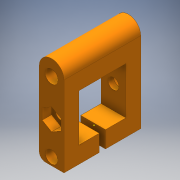
# Autodesk Inventor part: arm_grip
Saved by Autodesk Inventor 2016 (Build 200138000, 138)
## iProperties
Created: 2016-09-22
Part Number: arm_grip
Material: Nylon 6/6
Document SubType Name: Modeling
Designer: Jakub
Density: 1.13 g/cm^3
Appearance: Nylon 6
Mass: 4.12731 g
Surface Area: 27.5529 cm^2
Volume: 3.65248 cm^3
Author: Jakub
Autodesk Inventor part; units mm, degrees
ref_plane "YZ Plane" through (0, 0, 0) normal (1, 0, 0) x (0, 1, 0)
ref_plane "XZ Plane" through (0, 0, 0) normal (0, 1, 0) x (-1, 0, 0)
ref_plane "XY Plane" through (0, 0, 0) normal (0, 0, 1) x (1, 0, 0)
sketch "Sketch1" plane through (0, 0, 0) normal (1, 0, 0) x (0, 1, 0)
  line L0 (-12.4, 15) -> (12.4, 15)
  line L1 (12.4, 15) -> (12.4, -15)
  line L2 (12.4, -15) -> (-12.4, -15)
  line L3 (-12.4, -15) -> (-12.4, 15)
  line L4 (-12.4, 15) -> (12.4, -15) construction
  line L5 (12.4, 15) -> (-12.4, -15) construction
  line L6 (0, -15) -> (0, -1.5)
  circle A0 centre (0, -1.5) radius 8
  point P0 (0, 0)
  dimension "d0" = 24.8
  dimension "d1" = 30
  dimension "d2" = 13.5
  dimension "d3" = 16
  constraints: 14 end point, 3 midpoint, 2 parallel, 1 centre point, 1 coincident, 1 horizontal, 1 perpendicular, 1 vertical
  measures "d0" distance of L1.end L2.end
  measures "d1" distance of L0.end L1.end
  measures "d2" distance of L6.start L6.end
  measures "d3" diameter of A0
extrude "Extrusion1" add sketch "Sketch1" along normal blind 8
sketch "Sketch3" plane through (0, 12.4, 15) normal (0, 1, 0) x (1, 0, 0)
  line L0 (0, 0) -> (8, 0) projected
  line L1 (4, 0) -> (4, 5)
  circle A0 centre (4, 5) radius 2.1
  point P0 (0, 15)
  dimension "d9" = 5
  dimension "d10" = 4.2
  constraints: 2 end point, 1 centre point, 1 coincident, 1 midpoint, 1 vertical
  measures "d9" distance of L1.start L1.end
  measures "d10" diameter of A0
extrude "Extrusion3" cut sketch "Sketch3" against normal up to next
sketch "Sketch4" plane through (0, 12.4, 15) normal (0, 1, 0) x (1, 0, 0)
  line L0 (0, 30) -> (8, 30) projected
  line L1 (4, 30) -> (4, 27.5)
  circle A0 centre (4, 27.5) radius 1.25
  point P0 (0, 15)
  dimension "d13" = 2.5
  dimension "d14" = 2.5
  constraints: 2 end point, 1 centre point, 1 coincident, 1 midpoint, 1 vertical
  measures "d13" distance of L1.start L1.end
  measures "d14" diameter of A0
extrude "Extrusion4" cut sketch "Sketch4" against normal through all
fillet "Fillet1" radius 4 2 edges at (0, 0, 15) (8, 0, 15)
fillet "Fillet2" radius 2 1 edges at (0, 0, -15)
sketch "Sketch5" plane through (8, 0, 0) normal (1, 0, 0) x (0, 0, -1)
  arc A0 (1.5, 8) -> (1.5, 8) centre (1.5, 0) ccw projected
  circle A1 centre (1.5, 0) radius 8
  point P0 (0, 0)
  constraints: 1 centre point, 1 coincident
extrude "Extrusion5" add sketch "Sketch5" against normal blind 8
sketch "Sketch6" plane through (8, 0, 0) normal (1, 0, 0) x (0, 0, -1)
  line L0 (-5.6, -7.6) -> (9.6, -7.6)
  line L1 (9.6, -7.6) -> (9.6, 7.6)
  line L2 (9.6, 7.6) -> (-5.6, 7.6)
  line L3 (-5.6, 7.6) -> (-5.6, -7.6)
  line L4 (-5.6, -7.6) -> (9.6, 7.6) construction
  line L5 (9.6, -7.6) -> (-5.6, 7.6) construction
  point P0 (0, 0)
  point P1 (2, 0)
  dimension "d22" = 15.2
  dimension "d23" = 15.2
  dimension "d24" = 2
  constraints: 12 end point, 2 midpoint, 2 parallel, 1 horizontal, 1 perpendicular
  measures "d22" distance of L2.end L1.end
  measures "d23" distance of L1.end L0.end
  measures "d24" distance of point (0, 0) point (2, 0)
extrude "Extrusion6" cut sketch "Sketch6" against normal up to next
sketch "Sketch7" plane through (8, 0, 0) normal (1, 0, 0) x (0, 0, -1)
  line L0 (8.4724, -1) -> (16.4136, -1)
  line L1 (16.4136, -1) -> (16.4136, 1)
  line L2 (16.4136, 1) -> (8.4724, 1)
  line L3 (8.4724, 1) -> (8.4724, -1)
  line L4 (8.4724, -1) -> (16.4136, 1) construction
  line L5 (16.4136, -1) -> (8.4724, 1) construction
  point P0 (0, 0)
  point P1 (12.443, 0)
  dimension "d27" = 2
  constraints: 12 end point, 2 midpoint, 2 parallel, 1 horizontal, 1 perpendicular
  measures "d27" distance of L1.end L0.end
extrude "Extrusion7" cut sketch "Sketch7" against normal through all
sketch "Sketch8" plane through (4, 12.4, 11) normal (0, 1, 0) x (1, 0, 0)
  circle A0 centre (0, 23.5) radius 1.25 projected
  line L0 (0, 26) -> (2.1651, 24.75)
  line L1 (2.1651, 24.75) -> (2.1651, 22.25)
  line L2 (2.1651, 22.25) -> (0, 21)
  line L3 (0, 21) -> (-2.1651, 22.25)
  line L4 (-2.1651, 22.25) -> (-2.1651, 24.75)
  line L5 (-2.1651, 24.75) -> (0, 26)
  point P0 (-4, 11)
  dimension "d30" = 2.5
  constraints: 12 end point, 1 coincident, 13 other
  measures "d30" distance of L3.end L4.end
extrude "Extrusion8" cut sketch "Sketch8" against normal blind 8
sketch "Sketch9" plane through (4, 4.4, -10) normal (0.5, 0, -0.8660254) x (-0.8660254, 0, -0.5)
  point P0 (-1.5359, -4.4)
sketch "Sketch10" plane through (4, 12.4, 11) normal (0, 1, 0) x (1, 0, 0)
  line L0 (-2.1651, 24.75) -> (0, 26) projected
  line L1 (2.1651, 27.25) -> (-2.1651, 27.25)
  line L2 (-2.1651, 27.25) -> (-2.1651, 24.75)
  line L3 (-2.1651, 24.75) -> (2.1651, 24.75)
  line L4 (2.1651, 24.75) -> (2.1651, 27.25)
  line L5 (0, 26) -> (2.1651, 24.75) projected
  line L6 (2.1651, 27.25) -> (-2.1651, 24.75) construction
  line L7 (-2.1651, 27.25) -> (2.1651, 24.75) construction
  point P0 (-4, 11)
  constraints: 12 end point, 2 midpoint, 2 parallel, 1 horizontal, 1 perpendicular
extrude "Extrusion9" cut sketch "Sketch10" against normal blind 8
sketch "Sketch11" plane through (4, 12.4, 11) normal (0, 1, 0) x (1, 0, 0)
  line L0 (2.1651, 22.25) -> (0, 21) projected
  line L1 (0, 21) -> (-2.1651, 22.25)
  arc A0 (-2.1651, 25.9932) -> (-4, 24) centre (-2, 24) ccw projected
  line L2 (-4, 24) -> (-2.1651, 22.25)
  arc A1 (-2.1651, 25.9932) -> (-4, 24) centre (-2, 24) ccw
  line L3 (-2.1651, 25.9932) -> (2.1651, 26)
  line L4 (2.1651, 22.25) -> (0, 21) projected
  line L5 (2.1651, 26) -> (2.1651, 22.25)
  line L6 (2.1651, 22.25) -> (0, 21)
  circle A2 centre (0, 23.5) radius 1.25 projected
  circle A3 centre (0, 23.5) radius 1.25
  point P0 (-4, 11)
  constraints: 10 end point, 2 centre point, 2 point on circle, 1 coincident, 1 collinear, 1 concentric
extrude "Extrusion10" add sketch "Sketch11" against normal blind 5
sketch "Sketch12" plane through (4, -12.4, 11) normal (0, -1, 0) x (1, 0, 0)
  circle A0 centre (0, -23.5) radius 1.25 projected
  circle A1 centre (0, -23.5) radius 2
  point P0 (-4, -11)
  dimension "d37" = 4
  constraints: 1 centre point, 1 coincident
  measures "d37" diameter of A1
extrude "Extrusion11" cut sketch "Sketch12" against normal blind 4
sketch "Sketch13" plane through (4, 12.4, 11) normal (0, 1, 0) x (1, 0, 0)
  line L0 (-2, 26) -> (4, 26) projected
  line L1 (4, 26) -> (0, 26)
  line L2 (0, 26) -> (0, 13)
  line L3 (0, 13) -> (4, 13)
  line L4 (4, 13) -> (4, 26)
  circle A0 centre (0, 13) radius 1.75
  point P0 (-4, 11)
  dimension "d40" = 4
  dimension "d41" = 13
  dimension "d42" = 3.5
  constraints: 8 end point, 2 parallel, 1 centre point, 1 coincident, 1 horizontal, 1 perpendicular
  measures "d40" distance of L3.end L2.end
  measures "d41" distance of L2.end L1.end
  measures "d42" diameter of A0
extrude "Extrusion12" cut sketch "Sketch13" against normal through all contours A0 L3 L2 | L2 L3 A0
sketch "Sketch14" plane through (4, -12.4, 11) normal (0, -1, 0) x (1, 0, 0)
  circle A0 centre (0, -13) radius 1.75 projected
  line L0 (0, -16.5) -> (-3.0311, -14.75)
  line L1 (-3.0311, -14.75) -> (-3.0311, -11.25)
  line L2 (-3.0311, -11.25) -> (0, -9.5)
  line L3 (0, -9.5) -> (3.0311, -11.25)
  line L4 (3.0311, -11.25) -> (3.0311, -14.75)
  line L5 (3.0311, -14.75) -> (0, -16.5)
  point P0 (-4, -11)
  dimension "d45" = 3.5
  constraints: 12 end point, 1 coincident, 13 other
  measures "d45" distance of L3.end L4.end
extrude "Extrusion13" cut sketch "Sketch14" against normal blind 3
sketch "Sketch15" plane through (4, 12.4, 11) normal (0, 1, 0) x (1, 0, 0)
  circle A0 centre (0, 13) radius 1.75 projected
  circle A1 centre (0, 13) radius 3
  point P0 (-4, 11)
  dimension "d48" = 6
  constraints: 1 centre point, 1 coincident
  measures "d48" diameter of A1
extrude "Extrusion14" cut sketch "Sketch15" against normal blind 3
body "Solid1"
